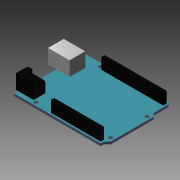
# Autodesk Inventor part: Arduino UNO
Saved by Autodesk Inventor 2015 (Build 190159000, 159)
## iProperties
Created: 2016-04-26
Part Number: Arduino UNO
Material: 一般
Document SubType Name: Modeling
Designer: yamashita1
Density: 1 g/cm^3
Appearance: 既定
Author: yamashita1
Autodesk Inventor part; units mm, degrees
ref_plane "YZ Plane" through (0, 0, 0) normal (1, 0, 0) x (0, 1, 0)
ref_plane "XZ Plane" through (0, 0, 0) normal (0, 1, 0) x (-1, 0, 0)
ref_plane "XY Plane" through (0, 0, 0) normal (0, 0, 1) x (1, 0, 0)
sketch "スケッチ1" plane through (0, 0, 0) normal (0, 0, 1) x (1, 0, 0)
  line L0 (0, 0) -> (66.04, 0)
  line L1 (66.04, 0) -> (66.04, 2.54)
  line L2 (66.04, 2.54) -> (68.58, 5.08)
  line L3 (68.58, 5.08) -> (68.58, 37.846)
  line L4 (68.58, 37.846) -> (66.04, 40.386)
  line L5 (66.04, 40.386) -> (66.04, 51.816)
  line L6 (66.04, 51.816) -> (64.516, 53.34)
  line L7 (64.516, 53.34) -> (0, 53.34)
  line L8 (0, 53.34) -> (0, 0)
  dimension "d0" = 66.04
  dimension "d1" = 2.54
  dimension "d2" = 2.54
  dimension "d3" = 2.54
  dimension "d4" = 32.766
  dimension "d5" = 2.54
  dimension "d6" = 2.54
  dimension "d7" = 11.43
  dimension "d8" = 1.524
  dimension "d9" = 1.524
  constraints: 18 end point, 3 vertical, 2 horizontal, 1 perpendicular
  measures "d0" distance of L0.start L0.end
  measures "d1" distance of L0.end L1.end
  measures "d2" horizontal distance of L2.end L1.end
  measures "d3" horizontal distance of L2.end L1.end
  measures "d4" distance of L2.end L3.end
  measures "d5" horizontal distance of L4.end L3.end
  measures "d6" horizontal distance of L4.end L3.end
  measures "d7" distance of L4.end L5.end
  measures "d8" horizontal distance of L6.end L5.end
  measures "d9" horizontal distance of L6.end L5.end
extrude "基板" add sketch "スケッチ1" along normal blind 1.8
sketch "スケッチ2" plane through (0, 0, 1.8) normal (0, 0, 1) x (1, 0, 0)
  circle A0 centre (13.97, 2.54) radius 1.5
  circle A1 centre (66.04, 7.62) radius 1.5
  circle A2 centre (66.04, 35.56) radius 1.5
  circle A3 centre (15.24, 50.8) radius 1.5
  point P0 (0, 0)
  dimension "d12" = 13.97
  dimension "d13" = 2.54
  dimension "d14" = 66.04
  dimension "d15" = 7.62
  dimension "d16" = 35.56
  dimension "d17" = 50.8
  dimension "d18" = 15.24
  dimension "d19" = 3
  constraints: 4 centre point, 4 coincident, 3 equal radius, 1 vertical alignment
  measures "d12" horizontal distance of point (13.97, 2.54) point (0, 0)
  measures "d13" vertical distance of point (13.97, 2.54) point (0, 0)
  measures "d14" horizontal distance of point (0, 0) point (66.04, 7.62)
  measures "d15" vertical distance of point (0, 0) point (66.04, 7.62)
  measures "d16" vertical distance of point (66.04, 35.56) point (0, 0)
  measures "d17" vertical distance of point (0, 0) point (15.24, 50.8)
  measures "d18" horizontal distance of point (0, 0) point (15.24, 50.8)
  measures "d19" diameter of A0
extrude "取付穴" cut sketch "スケッチ2" against normal blind 1.8
sketch "スケッチ4" plane through (0, 0, 1.8) normal (0, 0, 1) x (1, 0, 0)
  line L0 (11.595, 12.12) -> (-1.905, 12.12)
  line L1 (-1.905, 12.12) -> (-1.905, 3.12)
  line L2 (-1.905, 3.12) -> (11.595, 3.12)
  line L3 (11.595, 3.12) -> (11.595, 12.12)
  point P0 (0, 0)
  point P1 (-1.905, 7.62)
  point P2 (-1.905, 7.62)
  dimension "d22" = 7.62
  dimension "d23" = 1.905
  dimension "d24" = 13.5
  dimension "d25" = 9
  constraints: 8 end point, 2 coincident, 2 parallel, 1 horizontal, 1 midpoint, 1 perpendicular
  measures "d22" vertical distance of point (-1.905, 7.62) point (0, 0)
  measures "d23" horizontal distance of point (-1.905, 7.62) point (0, 0)
  measures "d24" distance of L2.end L1.end
  measures "d25" distance of L1.end L0.end
extrude "電源ジャック" add sketch "スケッチ4" along normal blind 11
sketch "スケッチ5" plane through (0, 0, 12.8) normal (0, 0, 1) x (1, 0, 0)
  line L0 (11.595, 12.12) -> (1.595, 12.12)
  line L1 (1.595, 12.12) -> (1.595, 3.12)
  line L2 (1.595, 3.12) -> (11.595, 3.12)
  line L3 (11.595, 3.12) -> (11.595, 12.12)
  line L4 (11.595, 3.12) -> (11.595, 12.12) projected
  point P0 (0, 0)
  point P1 (11.595, 7.62)
  dimension "d28" = 9
  dimension "d29" = 10
  constraints: 8 end point, 2 midpoint, 2 parallel, 1 horizontal, 1 perpendicular
  measures "d28" distance of L0.start L2.end
  measures "d29" distance of L1.end L2.end
extrude "押し出し4" cut sketch "スケッチ5" against normal blind 4.7
sketch "スケッチ6" plane through (0, 0, 8.1) normal (0, 0, 1) x (1, 0, 0)
  line L0 (11.595, 12.12) -> (1.595, 12.12)
  line L1 (1.595, 12.12) -> (1.595, 3.12)
  line L2 (1.595, 3.12) -> (11.595, 3.12)
  line L3 (11.595, 3.12) -> (11.595, 12.12)
  point P0 (0, 0)
  constraints: 8 end point, 2 parallel, 1 horizontal, 1 perpendicular
extrude "押し出し5" add sketch "スケッチ6" along normal blind 4.5
fillet "フィレット1" radius 4.5 2 edges at (6.595, 3.12, 12.6) (6.595, 12.12, 12.6)
sketch "スケッチ7" plane through (0, 0, 1.8) normal (0, 0, 1) x (1, 0, 0)
  line L0 (-6.35, 44.1) -> (10.05, 44.1)
  line L1 (10.05, 44.1) -> (10.05, 32.1)
  line L2 (10.05, 32.1) -> (-6.35, 32.1)
  line L3 (-6.35, 32.1) -> (-6.35, 44.1)
  point P0 (0, 0)
  point P1 (-6.35, 38.1)
  point P2 (-6.35, 38.1)
  dimension "d35" = 6.35
  dimension "d36" = 38.1
  dimension "d37" = 16.4
  dimension "d38" = 12
  constraints: 8 end point, 2 coincident, 2 parallel, 1 horizontal, 1 midpoint, 1 perpendicular
  measures "d35" horizontal distance of point (0, 0) point (-6.35, 38.1)
  measures "d36" vertical distance of point (0, 0) point (-6.35, 38.1)
  measures "d37" distance of L1.end L2.end
  measures "d38" distance of L0.end L1.end
extrude "USBジャック" add sketch "スケッチ7" along normal blind 11
sketch "スケッチ8" plane through (0, 0, 1.8) normal (0, 0, 1) x (1, 0, 0)
  line L0 (26.67, 3.81) -> (64.77, 3.81)
  line L1 (64.77, 3.81) -> (64.77, 1.27)
  line L2 (64.77, 1.27) -> (26.67, 1.27)
  line L3 (26.67, 1.27) -> (26.67, 3.81)
  point P0 (0, 0)
  point P1 (27.94, 2.54)
  point P2 (63.5, 2.54)
  point P3 (26.67, 2.54)
  dimension "d41" = 27.94
  dimension "d42" = 2.54
  dimension "d43" = 35.56
  dimension "d44" = 38.1
  dimension "d45" = 2.54
  dimension "d46" = 1.27
  constraints: 8 end point, 2 horizontal alignment, 2 parallel, 1 horizontal, 1 midpoint, 1 perpendicular
  measures "d41" horizontal distance of point (27.94, 2.54) point (0, 0)
  measures "d42" vertical distance of point (0, 0) point (27.94, 2.54)
  measures "d43" distance of point (63.5, 2.54) point (27.94, 2.54)
  measures "d44" distance of L0.end L0.start
  measures "d45" distance of L2.end L0.start
  measures "d46" distance of point (27.94, 2.54) point (26.67, 2.54)
extrude "POWER ANALOG IN" add sketch "スケッチ8" along normal blind 8.5
sketch "スケッチ9" plane through (0, 0, 1.8) normal (0, 0, 1) x (1, 0, 0)
  line L0 (17.526, 51.51) -> (64.77, 51.51)
  line L1 (64.77, 51.51) -> (64.77, 48.97)
  line L2 (64.77, 48.97) -> (17.526, 48.97)
  line L3 (17.526, 48.97) -> (17.526, 51.51)
  point P0 (0, 0)
  point P1 (18.796, 50.24)
  point P2 (63.5, 50.24)
  point P3 (17.526, 50.24)
  dimension "d49" = 50.24
  dimension "d50" = 18.796
  dimension "d51" = 44.704
  dimension "d52" = 2.54
  dimension "d53" = 47.244
  dimension "d54" = 1.27
  constraints: 8 end point, 2 horizontal alignment, 2 parallel, 1 horizontal, 1 midpoint, 1 perpendicular
  measures "d49" vertical distance of point (0, 0) point (18.796, 50.24)
  measures "d50" horizontal distance of point (0, 0) point (18.796, 50.24)
  measures "d51" distance of point (18.796, 50.24) point (63.5, 50.24)
  measures "d52" distance of L2.end L0.start
  measures "d53" distance of L1.end L2.end
  measures "d54" distance of point (18.796, 50.24) point (17.526, 50.24)
extrude "DIGITAL" add sketch "スケッチ9" along normal blind 8.5
